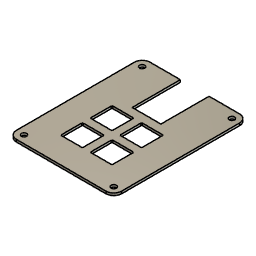
Cucu's Hackpad (Autodesk Fusion 360 archive; units mm, degrees)
design "HackPad Case"
Autodesk Fusion 360 part; units mm, degrees
sketch "Boceto1" plane through (0, 0, 0) normal (0, 1, 0) x (1, 0, 0)
  line L0 (3.025, -2.525) -> (16.025, -2.525)
  line L1 (3.025, -16.525) -> (16.025, -16.525)
  line L2 (2.525, -3.025) -> (2.525, -16.025)
  line L3 (16.525, -3.025) -> (16.525, -16.025)
  arc A0 (3.025, -2.525) -> (2.525, -3.025) centre (3.025, -3.025) ccw
  arc A1 (16.525, -3.025) -> (16.025, -2.525) centre (16.025, -3.025) ccw
  arc A2 (2.525, -16.025) -> (3.025, -16.525) centre (3.025, -16.025) ccw
  arc A3 (16.025, -16.525) -> (16.525, -16.025) centre (16.025, -16.025) ccw
  line L4 (22.075, -2.525) -> (35.075, -2.525)
  line L5 (22.075, -16.525) -> (35.075, -16.525)
  line L6 (21.575, -3.025) -> (21.575, -16.025)
  line L7 (35.575, -3.025) -> (35.575, -16.025)
  arc A4 (22.075, -2.525) -> (21.575, -3.025) centre (22.075, -3.025) ccw
  arc A5 (35.575, -3.025) -> (35.075, -2.525) centre (35.075, -3.025) ccw
  arc A6 (21.575, -16.025) -> (22.075, -16.525) centre (22.075, -16.025) ccw
  arc A7 (35.075, -16.525) -> (35.575, -16.025) centre (35.075, -16.025) ccw
  line L8 (3.025, -21.575) -> (16.025, -21.575)
  line L9 (3.025, -35.575) -> (16.025, -35.575)
  line L10 (2.525, -22.075) -> (2.525, -35.075)
  line L11 (16.525, -22.075) -> (16.525, -35.075)
  arc A8 (3.025, -21.575) -> (2.525, -22.075) centre (3.025, -22.075) ccw
  arc A9 (16.525, -22.075) -> (16.025, -21.575) centre (16.025, -22.075) ccw
  arc A10 (2.525, -35.075) -> (3.025, -35.575) centre (3.025, -35.075) ccw
  arc A11 (16.025, -35.575) -> (16.525, -35.075) centre (16.025, -35.075) ccw
  line L12 (22.075, -21.575) -> (35.075, -21.575)
  line L13 (22.075, -35.575) -> (35.075, -35.575)
  line L14 (21.575, -22.075) -> (21.575, -35.075)
  line L15 (35.575, -22.075) -> (35.575, -35.075)
  arc A12 (22.075, -21.575) -> (21.575, -22.075) centre (22.075, -22.075) ccw
  arc A13 (35.575, -22.075) -> (35.075, -21.575) centre (35.075, -22.075) ccw
  arc A14 (21.575, -35.075) -> (22.075, -35.575) centre (22.075, -35.075) ccw
  arc A15 (35.075, -35.575) -> (35.575, -35.075) centre (35.075, -35.075) ccw
  line L16 (-14.46, 33.91) -> (53.34, 33.91)
  line L17 (53.34, 33.91) -> (53.34, -52.19)
  line L18 (53.34, -52.19) -> (-14.46, -52.19)
  line L19 (-14.46, -52.19) -> (-14.46, 33.91)
  line L20 (10.09, 33.91) -> (28.59, 33.91)
  line L21 (28.59, 33.91) -> (28.59, 2.91)
  line L22 (28.59, 2.91) -> (10.09, 2.91)
  line L23 (10.09, 2.91) -> (10.09, 33.91)
  circle A16 centre (-9.46, 28.91) radius 1.7
  circle A17 centre (48.34, 28.91) radius 1.7
  circle A18 centre (-9.46, -47.19) radius 1.7
  circle A19 centre (48.34, -47.19) radius 1.7
  dimension "d1" = 86.1
  dimension "d2" = 67.8
  dimension "d3" = 16.615
  dimension "d4" = 16.985
  dimension "d5" = 17.765
  dimension "d6" = 18.5
  dimension "d7" = 31
  dimension "d8" = 24.55
  dimension "d9" = 3.4
  dimension "d10" = 3.4
  dimension "d11" = 3.4
  dimension "d12" = 3.4
  dimension "d13" = 5
  dimension "d14" = 5
  dimension "d15" = 5
  dimension "d16" = 5
  dimension "d17" = 5
  dimension "d18" = 5
  dimension "d19" = 5
  dimension "d20" = 5
  constraint horizontal L16
  constraint vertical L17
  constraint horizontal L18
  constraint vertical L19
  constraint horizontal L20
  constraint vertical L21
  constraint horizontal L22
  constraint vertical L23
  constraint coincident L16 L20.start
  measures "d1" distance of L16.start L18.end
  measures "d2" distance of L16.start L16.end
  measures "d3" distance of L9 L18
  measures "d4" distance of L10 L19
  measures "d5" distance of L7 L17
  measures "d6" distance of L20.start L20.end
  measures "d7" distance of L20.start L22.end
  measures "d8" distance of L19 L23
  measures "d9" diameter of A16
  measures "d10" diameter of A17
  measures "d11" diameter of A18
  measures "d12" diameter of A19
  measures "d13" distance of L16 A16.centre
  measures "d14" distance of L19 A16.centre
  measures "d15" distance of L16 A17.centre
  measures "d16" distance of L17 A17.centre
  measures "d17" distance of L17 A19.centre
  measures "d18" distance of L18 A19.centre
  measures "d19" distance of L18 A18.centre
  measures "d20" distance of L19 A18.centre
extrude "Extruir1" add sketch "Boceto1" along normal blind 1.5 contours L16 L17 L18 L19 L21 L22 L23
fillet "Empalme1" radius 5 4 edges at (-14.46, 0.75, 52.19) (53.34, 0.75, 52.19) (-14.46, 0.75, -33.91) (53.34, 0.75, -33.91)
